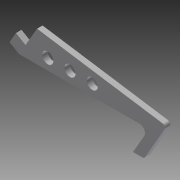
# Autodesk Inventor part: hook
Saved by Autodesk Inventor 2013 (Build 170138000, 138)
## iProperties
Created: 2013-01-20
Part Number: hook
Material: Steel
Document SubType Name: Modeling
Designer: Arpan
Density: 7.85 g/cm^3
Mass: 204.564 g
Surface Area: 118.434 cm^2
Volume: 26.0592 cm^3
Author: Arpan
Autodesk Inventor part; units mm, degrees
ref_plane "YZ Plane" through (0, 0, 0) normal (1, 0, 0) x (0, 1, 0)
ref_plane "XZ Plane" through (0, 0, 0) normal (0, 1, 0) x (-1, 0, 0)
ref_plane "XY Plane" through (0, 0, 0) normal (0, 0, 1) x (1, 0, 0)
sketch "Sketch1" plane through (0, 0, 0) normal (0, 0, 1) x (1, 0, 0)
  line L0 (0, 0) -> (130.048, 0)
  line L1 (87.9024, 12.7) -> (7.3323, 12.7)
  line L2 (87.9024, 12.7) -> (130.048, 12.7)
  line L3 (130.048, 12.7) -> (130.048, 0)
  line L4 (130.048, -31.75) -> (142.748, -31.75)
  line L5 (130.048, -31.75) -> (148.3789, 0)
  line L6 (142.748, -31.75) -> (168.4112, 12.7)
  line L7 (148.3789, 0) -> (130.048, 0)
  line L8 (130.048, 12.7) -> (168.4112, 12.7)
  line L9 (7.3323, 12.7) -> (-3.6662, 19.05)
  line L10 (-3.6662, 19.05) -> (-10.9985, 6.35)
  line L11 (-10.9985, 6.35) -> (0, 0)
  dimension "d4" = 130.048
  dimension "d7" = 31.75
  dimension "d8" = 12.7
  dimension "d9" = 60
  dimension "d10" = 60
  dimension "d11" = 12.7
  dimension "d14" = 12.7
  dimension "d15" = 10.9985
  dimension "d16" = 14.6647
  dimension "d17" = 150
  dimension "d18" = 150
  constraints: 24 end point, 3 perpendicular, 2 parallel, 1 collinear, 1 horizontal
  measures "d4" distance of L0.start L0.end
  measures "d7" distance of L0.end L4.start
  measures "d8" distance of L4.start L4.end
  measures "d9" angle of L5 L4
  measures "d10" angle of L4 L6
  measures "d11" distance between parallel lines of L1 L0
  measures "d14" distance of L1.end L9.end
  measures "d15" horizontal distance of L10.end L0.start
  measures "d16" distance of L9.end L10.end
  measures "d17" angle of L1 L9
  measures "d18" angle of L0 L11
extrude "Extrusion1" add sketch "Sketch1" along normal blind 6.35
sketch "Sketch2" plane through (0, 0, 6.35) normal (0, 0, 1) x (1, 0, 0)
  line L0 (168.4112, 12.7) -> (7.3323, 12.7) projected
  line L1 (-10.9985, 6.35) -> (0, 0) projected
  line L2 (7.3323, 12.7) -> (20.426, 35.379)
  line L3 (20.426, 35.379) -> (168.4112, 12.7)
  dimension "d19" = 26.1874
  constraints: 4 end point, 1 perpendicular
  measures "d19" distance of L0.end L2.end
extrude "Extrusion2" add sketch "Sketch2" against normal blind 6.35
fillet "Fillet1" radius 3.175 1 edges at (168.4112, 12.7, 3.175)
fillet "Fillet2" radius 3.175 1 edges at (142.748, -31.75, 3.175)
sketch "Sketch3" plane through (0, 0, 6.35) normal (0, 0, 1) x (1, 0, 0)
  circle A0 centre (32.7323, 12.7) radius 6.35
  circle A1 centre (58.1323, 12.7) radius 6.35
  circle A2 centre (83.5323, 12.7) radius 6.35
  dimension "d26" = 12.7
  dimension "d28" = 12.7
  dimension "d30" = 12.7
  constraints: 3 centre point
  measures "d26" diameter of A0
  measures "d28" diameter of A1
  measures "d30" diameter of A2
extrude "Extrusion3" cut sketch "Sketch3" against normal blind 6.35
fillet "Fillet4" radius 6.35 1 edges at (148.3789, 0, 3.175)
body "Solid1"
